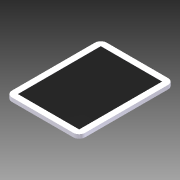
# Autodesk Inventor part: tablet
Saved by Autodesk Inventor 2012 SP1 (Build 160190100, 190)
## iProperties
Created: 2013-04-08
Part Number: tablet
Material: Default
Document SubType Name: Modeling
Designer: vogel
Density: 1 g/cm^3
Author: vogel
Autodesk Inventor part; units mm, degrees
ref_plane "YZ Plane" through (0, 0, 0) normal (1, 0, 0) x (0, 1, 0)
ref_plane "XZ Plane" through (0, 0, 0) normal (0, 1, 0) x (-1, 0, 0)
ref_plane "XY Plane" through (0, 0, 0) normal (0, 0, 1) x (1, 0, 0)
sketch "Skizze1" plane through (0, 0, 0) normal (0, 0, 1) x (1, 0, 0)
  line L0 (-93, 120.5) -> (93, 120.5)
  line L1 (93, 120.5) -> (93, -120.5)
  line L2 (93, -120.5) -> (-93, -120.5)
  line L3 (-93, -120.5) -> (-93, 120.5)
  line L4 (-130.2, 0) -> (130.2, 0) projected
  line L5 (0, -168.7) -> (0, 168.7) projected
  point P0 (0, 0)
  dimension "d0" = 241
  dimension "d1" = 186
  constraints: 8 end point, 2 parallel, 1 horizontal, 1 perpendicular, 2 other
  measures "d0" distance of L2.end L0.start
  measures "d1" distance of L1.end L2.end
extrude "Extrusion1" add sketch "Skizze1" along normal blind 10
sketch "Skizze3" plane through (0, 0, 10) normal (0, 0, 1) x (1, 0, 0)
  line L0 (93, 120.5) -> (93, -120.5) projected
  line L1 (-93, 120.5) -> (93, 120.5) projected
  line L2 (-93, -120.5) -> (-93, 120.5) projected
  line L3 (93, -120.5) -> (-93, -120.5) projected
  line L4 (78, 105.5) -> (78, -105.5)
  line L5 (78, -105.5) -> (-78, -105.5)
  line L6 (-78, -105.5) -> (-78, 105.5)
  line L7 (-78, 105.5) -> (78, 105.5)
  point P0 (0, 0)
  dimension "d5" = 15
  constraints: 8 end point, 3 other
  measures "d5" distance between parallel lines of L1 L7
extrude "Extrusion2" cut sketch "Skizze3" against normal blind 0.5 contours L4 L5 L6 L7
fillet "Rundung2" radius 15 4 edges at (-93, -120.5, 5) (93, -120.5, 5) (93, 120.5, 5) (-93, 120.5, 5)
